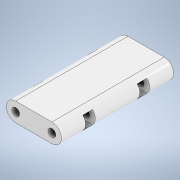
# Autodesk Inventor part: Standoff
Saved by Autodesk Inventor 2022 (Build 260153070, 153G)
## iProperties
Created: 2021-05-30
Part Number: Standoff
Material: PET Plastic
Document SubType Name: Modeling
Designer: elmar
Density: 1.541 g/cm^3
Appearance: White
Author: elmar
Autodesk Inventor part; units mm, degrees
ref_plane "YZ Plane" through (0, 0, 0) normal (1, 0, 0) x (0, 1, 0)
ref_plane "XZ Plane" through (0, 0, 0) normal (0, 1, 0) x (-1, 0, 0)
sketch "Sketch1" plane through (0, 0, 0) normal (0, 0, 1) x (1, 0, 0)
  line L0 (-7.5, 0) -> (7.5, 0) construction
  line L1 (-7.5, -3.9) -> (7.5, -3.9)
  line L2 (7.5, 3.9) -> (-7.5, 3.9)
  arc A0 (-7.5, 3.9) -> (-7.5, -3.9) centre (-7.5, 0) ccw
  arc A1 (7.5, -3.9) -> (7.5, 3.9) centre (7.5, 0) ccw
  point P0 (0, 0)
  point P1 (0, 0)
  dimension "d0" = 3.9
  dimension "d1" = 15
  constraints: 8 end point, 4 point on circle, 4 tangent, 2 centre point, 1 coincident, 1 horizontal, 1 midpoint, 1 parallel
  measures "d0" radius of A0
  measures "d1" distance of L0.start L0.end
extrude "Extrusion1" add sketch "Sketch1" along normal mid plane 46.5
sketch "Sketch2" plane through (0, 0, 23.25) normal (0, 0, 1) x (1, 0, 0)
  arc A0 (-7.5, 3.9) -> (-7.5, -3.9) centre (-7.5, 0) ccw projected
  arc A1 (7.5, -3.9) -> (7.5, 3.9) centre (7.5, 0) ccw projected
  point P0 (0, 0)
hole "Hole1" at (-7.5, 0, 23.25) at (7.5, 0, 23.25) direction (0, 0, -1) diameter 3.2 end through all clearance for "Flat Head Machine Screw" size "M3" standard "Ansi Metric M Profile"
ref_plane "Work Plane1" through (0, 0, 13.25) normal (0, 0, 1) x (1, 0, 0)
sketch "Sketch3" plane through (0, 0, 13.25) normal (0, 0, 1) x (1, 0, 0)
  circle A0 centre (-7.5, 0) radius 1.6 projected
  line L0 (-9.0877, 2.75) -> (-5.9123, 2.75)
  line L1 (-5.9123, 2.75) -> (-4.3246, 0)
  line L2 (-4.3246, 0) -> (-5.9123, -2.75)
  line L3 (-5.9123, -2.75) -> (-9.0877, -2.75)
  line L4 (-9.0877, -2.75) -> (-10.6754, 0)
  line L5 (-10.6754, 0) -> (-9.0877, 2.75)
  line L6 (-9.0877, 2.75) -> (-10.2654, 2.75)
  arc A1 (-7.5, 3.9) -> (-7.5, -3.9) centre (-7.5, 0) ccw projected
  line L7 (-9.0877, -2.75) -> (-10.2654, -2.75)
  point P0 (0, 0)
  dimension "d12" = 5.5
  constraints: 16 end point, 3 horizontal, 2 point on circle, 1 coincident, 13 other
  measures "d12" distance between parallel lines of L3 L0
extrude "Extrusion2" cut sketch "Sketch3" against normal blind 4
mirror "Mirror1" about plane through (0, 0, 0) normal (1, 0, 0) of "Extrusion2"
mirror "Mirror2" about plane through (0, 0, 0) normal (0, 0, 1) of "Extrusion2", "Mirror1"
body "Solid1"
